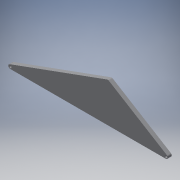
# Autodesk Inventor part: L3
Saved by Autodesk Inventor 2019 (Build 230136000, 136)
## iProperties
Created: 2020-03-18
Part Number: L3
Material: Generic
Document SubType Name: Modeling
Designer: Pulag
Density: 1 g/cm^3
Appearance: Default
Mass: 6.06377 g
Surface Area: 48.6603 cm^2
Volume: 6.06377 cm^3
Author: Pulag
Autodesk Inventor part; units mm, degrees
ref_plane "YZ Plane" through (0, 0, 0) normal (1, 0, 0) x (0, 1, 0)
ref_plane "XZ Plane" through (0, 0, 0) normal (0, 1, 0) x (-1, 0, 0)
ref_plane "XY Plane" through (0, 0, 0) normal (0, 0, 1) x (1, 0, 0)
sketch "Sketch1" plane through (0, 0, 0) normal (0, 0, 1) x (1, 0, 0)
  line L0 (0, 0) -> (120, 0)
  arc A0 (0, 3) -> (0, 0) centre (0, 1.5) ccw
  arc A1 (120, 0) -> (120, 3) centre (120, 1.5) ccw
  circle A2 centre (0, 1.5) radius 1
  circle A3 centre (120, 1.5) radius 1
  arc A4 (75.9569, 30.1419) -> (74.6624, 30.2712) centre (75.1754, 28.8616) ccw
  line L1 (53.292, 22.493) -> (62.7991, 25.9533)
  line L2 (62.7991, 25.9533) -> (74.6624, 30.2712)
  line L3 (53.292, 22.493) -> (-0.513, 2.9095)
  line L4 (80.4155, 27.4204) -> (88.5179, 22.4745)
  line L5 (80.4155, 27.4204) -> (75.9569, 30.1419)
  line L6 (88.5179, 22.4745) -> (120.7815, 2.7803)
  dimension "d0" = 2
  dimension "d1" = 2
  dimension "d2" = 120
  dimension "d8" = 3
  constraints: 14 end point, 8 point on circle, 5 centre point, 5 tangent, 2 coincident, 2 point on line, 1 horizontal
  measures "d0" diameter of A2
  measures "d1" diameter of A3
  measures "d2" distance of A1.centre A0.centre
  measures "d8" diameter of A4
extrude "Extrusion1" add sketch "Sketch1" along normal blind 3
body "Solid1"
